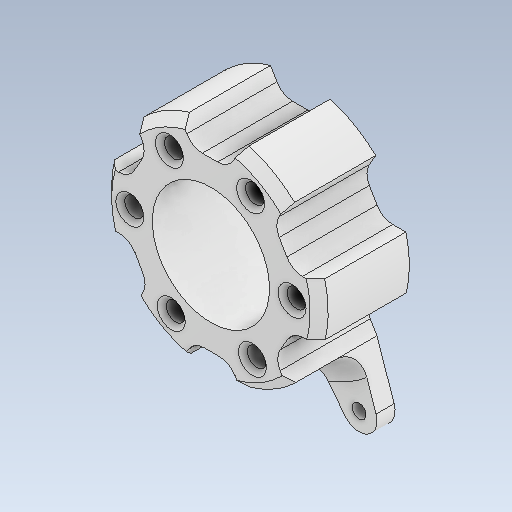
# Autodesk Inventor part: joint_connector_2
Saved by Autodesk Inventor 2020 (Build 240168000, 168)
## iProperties
Created: 2020-08-28
Part Number: joint_connector_2
Material: ABS Plastic
Document SubType Name: Modeling
Designer: psrobotics
Density: 1.06 g/cm^3
Appearance: Smooth - White
Author: psrobotics
Autodesk Inventor part; units mm, degrees
ref_plane "YZ Plane" through (0, 0, 0) normal (1, 0, 0) x (0, 1, 0)
ref_plane "XZ Plane" through (0, 0, 0) normal (0, 1, 0) x (-1, 0, 0)
ref_plane "XY Plane" through (0, 0, 0) normal (0, 0, 1) x (1, 0, 0)
sketch "Sketch1" plane through (0, 0, 0) normal (0, 0, 1) x (1, 0, 0)
  circle A0 centre (-69.978, 40.504) radius 13 projected
  arc A1 (-66.6416, 64.271) -> (-80.5887, 18.977) centre (-69.978, 40.504) ccw projected
  circle A2 centre (-61.1849, 56.2101) radius 2 projected
  circle A3 centre (-69.978, 40.504) radius 13
  circle A4 centre (-69.978, 40.504) radius 24
  circle A5 centre (-61.1849, 56.2101) radius 2.1
  circle A6 centre (-79.1833, 55.9721) radius 2.1
  circle A7 centre (-87.9764, 40.2661) radius 2.1
  circle A8 centre (-78.7712, 24.7979) radius 2.1
  circle A9 centre (-60.7727, 25.0359) radius 2.1
  circle A10 centre (-51.9796, 40.742) radius 2.1
  point P0 (0, 0)
  point P1 (-80.5887, 18.977)
  dimension "d0" = 26
  dimension "d1" = 48
  dimension "d2" = 4.2
  dimension "d5" = 360
  constraints: 8 centre point, 3 coincident, 13 other
  measures "d0" diameter of A3
  measures "d1" diameter of A4
  measures "d2" diameter of A5
extrude "Extrusion1" add sketch "Sketch1" along normal blind 20 contours A4 A1
sketch "Sketch2" plane through (-69.978, 40.504, 20) normal (0, 0, 1) x (1, 0, 0)
  circle A0 centre (0, 0) radius 24 projected
  circle A1 centre (0, 0) radius 13 projected
  circle A2 centre (8.7931, 15.7061) radius 2.1 projected
  circle A3 centre (-8.7931, -15.7061) radius 2.1 projected
  circle A4 centre (-17.9984, -0.238) radius 2.1 projected
  circle A5 centre (-9.2053, 15.4681) radius 2.1 projected
  circle A6 centre (9.2053, -15.4681) radius 2.1 projected
  circle A7 centre (17.9984, 0.238) radius 2.1 projected
  arc A8 (-15.3546, 10.5792) -> (-15.3546, 14.5792) centre (-18.8187, 12.5792) ccw projected
  line L0 (-16.8209, 17.1189) -> (-15.3546, 14.5792) projected
  line L1 (-15.3546, 10.5792) -> (-17.0452, 7.651) projected
  arc A9 (-20.5093, 5.651) -> (-17.0452, 7.651) centre (-20.5093, 9.651) ccw projected
  line L2 (-20.5093, 5.651) -> (-23.3252, 5.651) projected
  point P0 (69.978, -40.504)
extrude "Extrusion2" cut sketch "Sketch2" against normal blind 20 contours L0 A8 L1 A9 L2 A0 picked at (-18.9757, 11.386)
pattern_circular "Circular Pattern1" count 6 over 360 about axis through (-69.978, 40.504, 0) along (0, 0, 1) of "Extrusion2"
chamfer "Chamfer1" distance 1 angle 45 12 edges at (-54.0796, 40.742, 20) (-62.8727, 25.0359, 20) (-80.8712, 24.7979, 20) (-90.0764, 40.2661, 20) (-81.2833, 55.9721, 20) (-63.2849, 56.2101, 20) (-90.0764, 40.2661, 0) (-80.8712, 24.7979, 0) (-62.8727, 25.0359, 0) (-54.0796, 40.742, 0) (-63.2849, 56.2101, 0) (-81.2833, 55.9721, 0)
sketch "Sketch3" plane through (0, 0, 0) normal (0, 0, -1) x (-1, 0, 0)
  circle A0 centre (53.1186, 10.9547) radius 1.55 projected
  circle A1 centre (53.1186, 10.9547) radius 4
  circle A2 centre (79.1833, 55.9721) radius 3.1 projected
  circle A3 centre (78.7712, 24.7979) radius 3.1 projected
  circle A4 centre (51.9796, 40.742) radius 3.1 projected
  line L0 (75.3388, 61.0911) -> (76.7467, 63.5297) projected
  arc A5 (86.799, 57.6229) -> (76.7467, 63.5297) centre (69.978, 40.504) ccw projected
  line L1 (86.799, 57.6229) -> (85.3327, 55.0832) projected
  arc A6 (85.3327, 55.0832) -> (85.3327, 51.0832) centre (88.7968, 53.0832) ccw projected
  line L2 (85.3327, 51.0832) -> (87.0233, 48.155) projected
  arc A7 (87.0233, 48.155) -> (90.4874, 46.155) centre (90.4874, 50.155) ccw projected
  line L3 (90.4874, 46.155) -> (93.3032, 46.155) projected
  arc A8 (93.2139, 34.4961) -> (93.3032, 46.155) centre (69.978, 40.504) ccw projected
  line L4 (93.2139, 34.4961) -> (90.2813, 34.4961) projected
  arc A9 (90.2813, 34.4961) -> (86.8172, 32.4961) centre (90.2813, 30.4961) ccw projected
  line L5 (86.8172, 32.4961) -> (85.1266, 29.5679) projected
  arc A10 (85.1266, 29.5679) -> (85.1266, 25.5679) centre (88.5907, 27.5679) ccw projected
  line L6 (85.1266, 25.5679) -> (86.5345, 23.1293) projected
  arc A11 (76.3929, 17.3772) -> (86.5345, 23.1293) centre (69.978, 40.504) ccw projected
  line L7 (76.3929, 17.3772) -> (74.9266, 19.9169) projected
  arc A12 (74.9266, 19.9169) -> (71.4625, 21.9169) centre (71.4625, 17.9169) ccw projected
  line L8 (71.4625, 21.9169) -> (68.0813, 21.9169) projected
  arc A13 (68.0813, 21.9169) -> (64.6172, 19.9169) centre (68.0813, 17.9169) ccw projected
  line L9 (64.6172, 19.9169) -> (63.2093, 17.4783) projected
  arc A14 (53.1571, 23.3851) -> (63.2093, 17.4783) centre (69.978, 40.504) ccw projected
  line L10 (53.1571, 23.3851) -> (54.6234, 25.9248) projected
  arc A15 (54.6234, 25.9248) -> (54.6234, 29.9248) centre (51.1593, 27.9248) ccw projected
  line L11 (54.6234, 29.9248) -> (52.9328, 32.853) projected
  arc A16 (52.9328, 32.853) -> (49.4687, 34.853) centre (49.4687, 30.853) ccw projected
  line L12 (49.4687, 34.853) -> (46.6528, 34.853) projected
  arc A17 (46.7422, 46.5119) -> (46.6528, 34.853) centre (69.978, 40.504) ccw projected
  line L13 (46.7422, 46.5119) -> (49.6748, 46.5119) projected
  arc A18 (49.6748, 46.5119) -> (53.1389, 48.5119) centre (49.6748, 50.5119) ccw projected
  line L14 (53.1389, 48.5119) -> (54.8295, 51.4401) projected
  arc A19 (54.8295, 51.4401) -> (54.8295, 55.4401) centre (51.3654, 53.4401) ccw projected
  line L15 (54.8295, 55.4401) -> (53.4215, 57.8788) projected
  arc A20 (63.5631, 63.6308) -> (53.4215, 57.8788) centre (69.978, 40.504) ccw projected
  line L16 (63.5631, 63.6308) -> (65.0294, 61.0911) projected
  arc A21 (65.0294, 61.0911) -> (68.4935, 59.0911) centre (68.4935, 63.0911) ccw projected
  line L17 (68.4935, 59.0911) -> (71.8747, 59.0911) projected
  arc A22 (71.8747, 59.0911) -> (75.3388, 61.0911) centre (71.8747, 63.0911) ccw projected
  circle A23 centre (69.978, 40.504) radius 13 projected
  circle A24 centre (60.7727, 25.0359) radius 3.1 projected
  circle A25 centre (87.9764, 40.2661) radius 3.1 projected
  circle A26 centre (61.1849, 56.2101) radius 3.1 projected
  line L18 (53.1571, 23.3851) -> (49.3354, 12.2536)
  line L19 (63.2093, 17.4783) -> (64.6172, 19.9169) projected
  line L20 (63.2093, 17.4783) -> (56.2847, 8.5101)
  point P0 (0, 0)
  dimension "d17" = 8
  constraints: 4 end point, 2 point on circle, 2 tangent, 1 centre point, 1 coincident
  measures "d17" diameter of A1
extrude "Extrusion3" add sketch "Sketch3" against normal blind 4 contours A1 | A1 L18 A14 L20
fillet "Fillet1" radius 5 1 edges at (-57.819, 19.812, 4)
chamfer "Chamfer2" distance 2 angle 45 6 edges at (-82.137, 61.196, 20) (-58.1377, 61.38, 20) (-45.9787, 40.688, 20) (-57.819, 19.812, 20) (-81.8183, 19.628, 20) (-93.9773, 40.32, 20)
body "Solid1"
